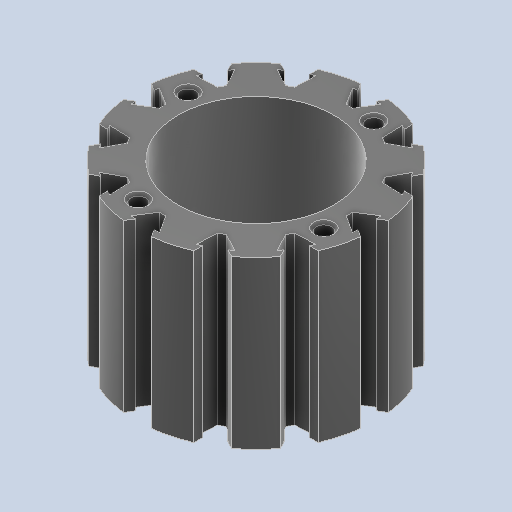
# Autodesk Inventor part: rotor_plastic
Saved by Autodesk Inventor 2025 (Build 290162000, 162)
## iProperties
Created: 2026-08-03
Part Number: rotor_plastic
Material: Ogólny
Document SubType Name: Modeling
Designer: zzapa
Density: 1 g/cm^3
Appearance: Gładki — czarny
Author: zzapa
Autodesk Inventor part; units mm, degrees
ref_plane "YZ Plane" through (0, 0, 0) normal (1, 0, 0) x (0, 1, 0)
ref_plane "XZ Plane" through (0, 0, 0) normal (0, 1, 0) x (-1, 0, 0)
ref_plane "XY Plane" through (0, 0, 0) normal (0, 0, 1) x (1, 0, 0)
sketch "Szkic1" plane through (0, 0, 0) normal (0, 1, 0) x (-1, 0, 0)
  circle A0 centre (0, 0) radius 23
  circle A1 centre (0, 0) radius 15
  line L0 (32.2, 0) -> (-32.2, 0) projected
  line L1 (0, -32.2) -> (0, 32.2) projected
  line L2 (-22.7168, -3.598) -> (-17, 0)
  line L3 (-22.7168, 3.598) -> (-17, 0)
  line L4 (0, 0) -> (-22.7168, -3.598)
  circle A2 centre (0, 0) radius 18
  line L5 (-17.9892, 0.6226) -> (-22.7168, 3.598)
  line L6 (-17.9892, -0.6226) -> (-22.7168, -3.598)
  line L7 (-15.8904, -8.4554) -> (-21.4723, -8.2425)
  line L8 (-15.2678, -9.5338) -> (-17.8744, -14.4744)
  line L9 (-9.5338, -15.2678) -> (-14.4744, -17.8744)
  line L10 (-8.4554, -15.8904) -> (-8.2425, -21.4723)
  line L11 (-0.6226, -17.9892) -> (-3.598, -22.7168)
  line L12 (0.6226, -17.9892) -> (3.598, -22.7168)
  line L13 (8.4554, -15.8904) -> (8.2425, -21.4723)
  line L14 (9.5338, -15.2678) -> (14.4744, -17.8744)
  line L15 (15.2678, -9.5338) -> (17.8744, -14.4744)
  line L16 (15.8904, -8.4554) -> (21.4723, -8.2425)
  line L17 (17.9892, -0.6226) -> (22.7168, -3.598)
  line L18 (17.9892, 0.6226) -> (22.7168, 3.598)
  line L19 (15.8904, 8.4554) -> (21.4723, 8.2425)
  line L20 (15.2678, 9.5338) -> (17.8744, 14.4744)
  line L21 (9.5338, 15.2678) -> (14.4744, 17.8744)
  line L22 (8.4554, 15.8904) -> (8.2425, 21.4723)
  line L23 (0.6226, 17.9892) -> (3.598, 22.7168)
  line L24 (-0.6226, 17.9892) -> (-3.598, 22.7168)
  line L25 (-8.4554, 15.8904) -> (-8.2425, 21.4723)
  line L26 (-9.5338, 15.2678) -> (-14.4744, 17.8744)
  line L27 (-15.2678, 9.5338) -> (-17.8744, 14.4744)
  line L28 (-15.8904, 8.4554) -> (-21.4723, 8.2425)
  dimension "d0" = 46
  dimension "d9" = 36
  dimension "d1" = 30
  dimension "d2" = 17
  dimension "d4" = 9
  dimension "d12" = 360
  constraints: 54 end point, 4 point on line, 3 coincident, 2 collinear, 1 centre point, 1 symmetric about line, 93 other
  measures "d1" diameter of A1
  measures "d2" distance of L2.end point (0, 0)
  measures "d4" angle of L4 L0
extrude "Wyciągnięcie proste1" add sketch "Szkic1" along normal blind 32 contours L18 A2 L19 A0 | A0 L16 A2 L17 | A2 L1 A1 L0 | L0 A1 L1 A2 | L20 A2 L21 A0 | A0 L14 A2 L15 | A1 L0 L3 A2 L1 | L1 A2 L4 A1 | A1 L4 A2 L2 L0 | L22 A2 L23 A0 | A0 L12 A2 L13 | L2 A2 L0 | L0 A2 L3 | A2 L25 A0 L24 | A2 L7 A0 L4 | L4 L2 A2 | L11 A0 L10 A2 | L3 A0 L28 A2 | A2 L27 A0 L26 | A2 L9 A0 L8
sketch "Szkic2" plane through (0, 32, 0) normal (0, 1, 0) x (1, 0, 0)
  arc A0 (-17.8744, -14.4744) -> (-14.4744, -17.8744) centre (0, 0) ccw projected
  circle A1 centre (0, 0) radius 23
  circle A2 centre (0, 0) radius 21.5
  line L0 (22.7168, -3.598) -> (17.9892, -0.6226) projected
  line L1 (17.9892, 0.6226) -> (22.7168, 3.598) projected
  line L2 (22.8434, -2.679) -> (21.4256, -1.7867)
  line L3 (-32.2, 0) -> (32.2, 0) projected
  arc A3 (21.4723, -8.2425) -> (22.7168, -3.598) centre (0, 0) ccw projected
  line L4 (0, 0) -> (22.2163, -5.9528)
  arc A4 (21.4723, -8.2425) -> (22.7168, -3.598) centre (0, 0) ccw projected
  line L5 (21.1225, -9.1016) -> (19.4485, -9.1655)
  line L6 (22.8434, 2.679) -> (21.4256, 1.7867)
  line L7 (21.1225, 9.1016) -> (19.4485, 9.1655)
  line L8 (18.4435, 13.7418) -> (17.6618, 12.2601)
  line L9 (13.7418, 18.4435) -> (12.2601, 17.6618)
  line L10 (9.1016, 21.1225) -> (9.1655, 19.4485)
  line L11 (2.679, 22.8434) -> (1.7867, 21.4256)
  line L12 (-2.679, 22.8434) -> (-1.7867, 21.4256)
  line L13 (-9.1016, 21.1225) -> (-9.1655, 19.4485)
  line L14 (-13.7418, 18.4435) -> (-12.2601, 17.6618)
  line L15 (-18.4435, 13.7418) -> (-17.6618, 12.2601)
  line L16 (-21.1225, 9.1016) -> (-19.4485, 9.1655)
  line L17 (-22.8434, 2.679) -> (-21.4256, 1.7867)
  line L18 (-22.8434, -2.679) -> (-21.4256, -1.7867)
  line L19 (-21.1225, -9.1016) -> (-19.4485, -9.1655)
  line L20 (-18.4435, -13.7418) -> (-17.6618, -12.2601)
  line L21 (-13.7418, -18.4435) -> (-12.2601, -17.6618)
  line L22 (-9.1016, -21.1225) -> (-9.1655, -19.4485)
  line L23 (-2.679, -22.8434) -> (-1.7867, -21.4256)
  line L24 (2.679, -22.8434) -> (1.7867, -21.4256)
  line L25 (9.1016, -21.1225) -> (9.1655, -19.4485)
  line L26 (13.7418, -18.4435) -> (12.2601, -17.6618)
  line L27 (18.4435, -13.7418) -> (17.6618, -12.2601)
  point P0 (21.4256, 1.7867)
  point P1 (22.8434, 2.679)
  point P2 (21.1225, 9.1016)
  point P3 (19.4485, 9.1655)
  point P4 (19.4485, -9.1655)
  point P5 (21.1225, -9.1016)
  point P6 (13.7418, 18.4435)
  point P7 (12.2601, 17.6618)
  point P8 (17.6618, 12.2601)
  point P9 (18.4435, 13.7418)
  point P10 (2.679, 22.8434)
  point P11 (1.7867, 21.4256)
  point P12 (9.1655, 19.4485)
  point P13 (9.1016, 21.1225)
  point P14 (-9.1016, 21.1225)
  point P15 (-9.1655, 19.4485)
  point P16 (-1.7867, 21.4256)
  point P17 (-2.679, 22.8434)
  point P18 (-17.6618, 12.2601)
  point P19 (-12.2601, 17.6618)
  point P20 (-13.7418, 18.4435)
  point P21 (-22.8434, 2.679)
  point P22 (-21.4256, 1.7867)
  point P23 (-19.4485, 9.1655)
  point P24 (-21.1225, 9.1016)
  point P25 (-21.1225, -9.1016)
  point P26 (-19.4485, -9.1655)
  point P27 (-21.4256, -1.7867)
  point P28 (-22.8434, -2.679)
  point P29 (-13.7418, -18.4435)
  point P30 (-12.2601, -17.6618)
  point P31 (-17.6618, -12.2601)
  point P32 (-18.4435, -13.7418)
  point P33 (-17.8744, -14.4744)
  point P34 (-14.4744, -17.8744)
  point P35 (-2.679, -22.8434)
  point P36 (-1.7867, -21.4256)
  point P37 (-9.1655, -19.4485)
  point P38 (-9.1016, -21.1225)
  point P39 (9.1016, -21.1225)
  point P40 (9.1655, -19.4485)
  point P41 (1.7867, -21.4256)
  point P42 (2.679, -22.8434)
  point P43 (17.6618, -12.2601)
  point P44 (12.2601, -17.6618)
  dimension "d16" = 1.5
  dimension "d19" = 360
  constraints: 50 end point, 2 coincident, 2 point on circle, 2 symmetric about line, 1 parallel, 80 other
extrude "Wyciągnięcie proste2" add sketch "Szkic2" against normal up to surface (32 mm away) contours A1 L20 A2 L21 A0 | A1 L18 A2 L19 | L22 A2 L23 A1 | L24 A2 L25 A1 | A1 L16 A2 L17 | L26 A2 L27 A1 | A1 L14 A2 L15 | L4 A1 L5 A2 | A2 L0 A1 L4 | A2 L1 A1 L6 | L2 A1 L0 A2 | A1 L12 A2 L13 | A2 L7 A1 L1 | A1 L10 A2 L11 | A2 L9 A1 L8
sketch "Szkic3" plane through (0, 32, 0) normal (0, 1, 0) x (1, 0, 0)
  arc A0 (-9.1016, -21.1225) -> (-2.679, -22.8434) centre (0, 0) ccw projected
  line L0 (-5.9528, -22.2163) -> (0, 0)
  circle A1 centre (0, 0) radius 18.5
  point P0 (-4.7882, -17.8696)
  point P1 (17.8696, -4.7882)
  point P2 (4.7882, 17.8696)
  point P3 (-17.8696, 4.7882)
  dimension "d27" = 37
  dimension "d25" = 360
  constraints: 2 end point, 1 coincident, 1 point on circle, 1 point on line, 8 other
hole "Otwór1" at (-4.7882, 32, 17.8696) at (17.8696, 32, 4.7882) at (4.7882, 32, -17.8696) at (-17.8696, 32, -4.7882) direction (0, -1, 0) diameter 2.9 depth 7
ref_plane "Płaszczyzna konstrukcyjna1" through (0, 16, 0) normal (0, -1, 0) x (1, 0, 0)
mirror "Odbij1" about plane through (0, 16, 0) normal (0, -1, 0) of "Otwór1"
chamfer "Faza2" distance 0.5 angle 45 8 edges at (4.7882, 32, -19.3196) (17.8696, 32, 3.3382) (-4.7882, 32, 16.4196) (-17.8696, 32, -6.2382) (-4.7882, 0, 16.4196) (17.8696, 0, 3.3382) (4.7882, 0, -19.3196) (-17.8696, 0, -6.2382)
ref_plane "Płaszczyzna konstrukcyjna2" through (-14.7224, 0, 8.5) normal (0.5, 0, 0.8660254) x (0, 1, 0)
equation "\"d0\" = 2 * rotor_out_r"
equation "\"d9\" = 2 * rotor_coil_groove_in_correction_r"
equation "\"d1\" = 2 * rotor_core_r"
equation "\"d2\" = rotor_coil_groove_in_r"
equation "\"d4\" = 0.5 * rotor_coil_groove_ang"
equation "\"d14\" = rotor_plastic_h"
equation "\"d16\" = rotor_teeth_d"
equation "\"d21\" = rotor_plastic_h"
equation "\"d27\" = rotor_plastic_insert_r"
equation "\"d28\" = insert_m2_d"
equation "\"d33\" = insert_m2_h"
equation "\"d38\" = insert25m_corner"
equation "\"stator_out_d\" = 2.5"
equation "\"stator_h\" = 45"
equation "\"mag_size_x\" = 7"
equation "\"mag_size_y\" = 3"
equation "\"mag_corner_r\" = 0.4"
equation "\"magnet_ring_r\" = 27.5"
equation "\"magnet_ring_d\" = 3.3"
equation "\"magnet_ring_h\" = 36"
equation "\"magnet_ring_pocket_mag_size_x\" = 7.1"
equation "\"magnet_ring_pocket_mag_size_y\" = 3.1"
equation "\"magnet_ring_pocket_mag_size_z\" = 10.3"
equation "\"magnet_ring_pocket_radial_cut\" = 1.4"
equation "\"casing_d\" = 3"
equation "\"rotor_out_r\" = 23"
equation "\"rotor_coil_groove_in_r\" = 17"
equation "\"rotor_core_r\" = 15"
equation "\"rotor_coil_groove_ang\" = 18deg"
equation "\"rotor_coil_groove_in_correction_r\" = 18"
equation "\"rotor_plastic_h\" = 32"
equation "\"rotor_teeth_d\" = 1.5"
equation "\"shaft_d\" = 8"
equation "\"insert25m_d\" = 2.9"
equation "\"insert25m_corner\" = 0.5"
equation "\"insert25m_h\" = 7"
equation "\"rotor_plastic_insert_r\" = 37"
equation "\"shaft_lock_1_d\" = 8"
equation "\"shaf_lock_1_D\" = 32"
equation "\"shaft_lock_1_D\" = 44"
equation "\"shaft_lock_1_h1\" = 3.5"
equation "\"shaft_lock_1_insert_part_h\" = 8"
equation "\"shaft_lock_1_corner\" = 2"
equation "\"shaft_lock_1_insert_part_a\" = 18"
equation "\"shaft_lock_2_h1\" = 3.5"
equation "\"shaft_lock_2_d\" = 8"
equation "\"shaft_lock_2_insert_part_a\" = 18"
equation "\"shaft_lock_2_D\" = 44"
equation "\"shaft_lock_2_corner\" = 2"
equation "\"shaft_lock_2_insert_part_h\" = 7"
equation "\"shaft_lock_2_rotor_insert_grove_d_in\" = 36"
equation "\"shaft_lock_2_rotor_insert_grove_width_out\" = 5.5"
equation "\"shaft_lock_2_rotor_insert_grove_width_in\" = 7.6"
equation "\"shaft_lock_2_rotor_insert_r\" = 37"
equation "\"shaft_lock_2_rotor_insert_screw_d\" = 2.6"
equation "\"insert25m_pocket_d\" = 2.6"
equation "\"insert25m_pocket_D\" = 4.5"
equation "\"insert25m_pocket_nut_h\" = 1.5"
equation "\"insert_m2_pocket_d\" = 2.6"
equation "\"insert_m2_h\" = 7"
equation "\"insert_m2_d\" = 2.9"
equation "\"insert_m2_corner\" = 0.5"
equation "\"insert_m2_pocket_D\" = 4.5"
equation "\"insert_m2_pocket_nut_h\" = 1.5"
equation "\"shaft_lock_1_insert_part_corner\" = 6"
equation "\"shaft_lock_1_insert_part_pos\" = 4"
equation "\"shaft_lock_1_rotor_insert_grove_width_in\" = 7.6"
equation "\"shaft_lock_1_rotor_insert_r\" = 37"
equation "\"shaft_lock_1_rotor_insert_grove_d_in\" = 36"
equation "\"shaft_lock_1_rotor_insert_grove_width_out\" = 5.5"
equation "\"shaft_lock_1_shaft_insert_axial_cut_out_width\" = 12"
equation "\"shaft_lock_1_shaft_insert_axial_cut_in_width\" = 5.4"
equation "\"shaft_lock_1_shaft_insert_corner\" = 2"
equation "\"shaft_lock_1_shaft_insert_corner_finish\" = 0.5"
equation "\"shaft_lock_1_shaft_insert_pos\" = 2.5"
equation "\"shaft_lock_2_shaft_insert_corner\" = 2"
equation "\"shaft_lock_2_shaft_insert_pos\" = 2.5"
equation "\"shaft_lock_2_shaft_insert_axial_cut_in_width\" = 5.4"
equation "\"shaft_lock_2_shaft_insert_axial_cut_out_width\" = 12"
equation "\"shaft_lock_2_shaft_insert_corner_finish\" = 0.5"
equation "\"commutator_plate_D\" = 22"
equation "\"commutator_plastic_d\" = 1"
equation "\"commutator_plastic_h\" = 15"
equation "\"commutator_plate_ang\" = 55deg"
equation "\"commutator_plate_d\" = 1"
equation "\"commutator_plate_h\" = 15"
equation "\"commutator_plastic_shaft_d\" = 8"
equation "\"commutator_plastic_insert_cut_deepness\" = 1"
equation "\"commutator_plastic_insert_cut_length\" = 6"
equation "\"commutator_plastic_insert_pos\" = 3"
equation "\"commutator_plate_insert_pos\" = 3"
equation "\"casing_lock_hole_r\" = 14"
equation "\"casing_lock_h\" = 8"
equation "\"casing_stator_fix_r\" = 23"
equation "\"casing_stator_fix_h\" = 6"
equation "\"magnet_ring_insert_part_lengthen\" = 8"
equation "\"casing_sidebar_length\" = 3"
equation "\"casing_vent_hole_length\" = 4"
equation "\"casing_vent_hole_width\" = 7"
equation "\"sleeve_cup_r\" = 22"
equation "\"sleeve_cup_h\" = 3"
equation "\"sleeve_d\" = 3"
equation "\"sleeve_in_r\" = 11"
equation "\"casing_head_insert_r\" = 19"
equation "\"sleeve_head_insert_r\" = 19"
equation "\"magnet_ring_insert_part_radius_cut\" = 0.17"
equation "\"magnet_ring_insert_part_axial_flat_cut\" = 0.17"
equation "\"magnet_ring_insert_pos\" = 4"
equation "\"casing_radial_stator_insert_pos\" = 18.1"
equation "\"stator_radial_screw_d\" = 4"
equation "\"stator_radial_screw_pos\" = 4"
equation "\"rotor_sleeve_out_D\" = 10.5"
equation "\"rotor_sleeve_in_D\" = 8"
equation "\"rotor_sleeve_h\" = 32"
equation "\"carbon_brush_batt_d\" = 5"
